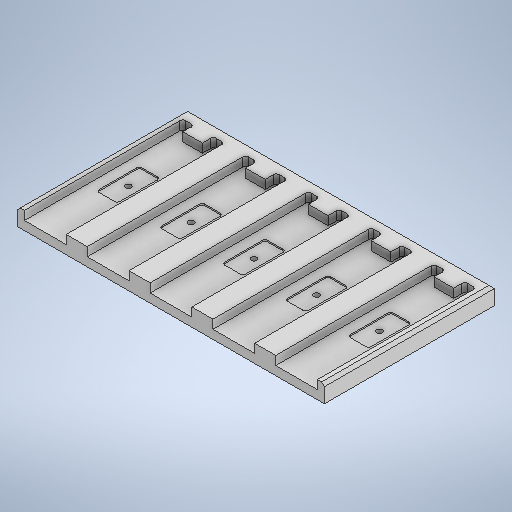
# Autodesk Inventor part: CROC Wirebonding Plate
Saved by Autodesk Inventor 2025 (Build 290162000, 162)
## iProperties
Created: 2025-05-07
Part Number: CROC Wirebonding Plate
Material: Generic
Document SubType Name: Modeling
Designer: Caleb Fangmeier
Density: 1 g/cm^3
Appearance: Default
Author: Caleb Fangmeier
Autodesk Inventor part; units mm, degrees
ref_plane "YZ Plane" through (0, 0, 0) normal (1, 0, 0) x (0, 1, 0)
ref_plane "XZ Plane" through (0, 0, 0) normal (0, 1, 0) x (-1, 0, 0)
ref_plane "XY Plane" through (0, 0, 0) normal (0, 0, 1) x (1, 0, 0)
sketch "Sketch1" plane through (0, 0, 0) normal (0, 1, 0) x (-1, 0, 0)
  line L0 (-111, 61.5) -> (111, 61.5)
  line L1 (111, 61.5) -> (111, -61.5)
  line L2 (111, -61.5) -> (-111, -61.5)
  line L3 (-111, -61.5) -> (-111, 61.5)
  line L4 (-111, 61.5) -> (111, -61.5) construction
  line L5 (111, 61.5) -> (-111, -61.5) construction
  point P0 (0, 0)
  dimension "d0" = 222
  dimension "d1" = 123
  constraints: 12 end point, 2 midpoint, 2 parallel, 1 horizontal, 1 perpendicular
  measures "d0" distance of L1.end L2.end
  measures "d1" distance of L0.end L1.end
extrude "Extrusion1" add sketch "Sketch1" along normal blind 12.7
sketch "Sketch2" plane through (0, 12.7, 0) normal (0, 1, 0) x (1, 0, 0)
  line L0 (-111, -61.5) -> (111, -61.5) projected
  line L1 (-106, -61.5) -> (-75.8, -61.5)
  line L2 (-75.8, -61.5) -> (-75.8, 45)
  line L3 (-75.8, 45) -> (-106, 45)
  line L4 (-106, 45) -> (-106, -61.5)
  line L5 (-111, 61.5) -> (-111, -61.5) projected
  line L6 (-106, 45) -> (-98, 45)
  line L7 (-98, 45) -> (-98, 51)
  line L8 (-100, 53) -> (-104, 53)
  line L9 (-106, 51) -> (-106, 45)
  line L10 (-75.8, 45) -> (-83.8, 45)
  line L11 (-83.8, 45) -> (-83.8, 51)
  line L12 (-81.8, 53) -> (-77.8, 53)
  line L13 (-75.8, 51) -> (-75.8, 45)
  arc A0 (-104, 53) -> (-106, 51) centre (-104, 51) ccw
  arc A1 (-98, 51) -> (-100, 53) centre (-100, 51) ccw
  arc A2 (-81.8, 53) -> (-83.8, 51) centre (-81.8, 51) ccw
  arc A3 (-75.8, 51) -> (-77.8, 53) centre (-77.8, 51) ccw
  line L14 (-60.55, -61.5) -> (-30.35, -61.5)
  line L15 (-30.35, -61.5) -> (-30.35, 45)
  arc A4 (-58.55, 53) -> (-60.55, 51) centre (-58.55, 51) ccw
  line L16 (-60.55, 51) -> (-60.55, 45)
  line L17 (-60.55, 45) -> (-60.55, -61.5)
  line L18 (-30.35, 45) -> (-60.55, 45)
  line L19 (-60.55, 45) -> (-52.55, 45)
  line L20 (-54.55, 53) -> (-58.55, 53)
  line L21 (-52.55, 45) -> (-52.55, 51)
  arc A5 (-52.55, 51) -> (-54.55, 53) centre (-54.55, 51) ccw
  line L22 (-38.35, 45) -> (-38.35, 51)
  arc A6 (-36.35, 53) -> (-38.35, 51) centre (-36.35, 51) ccw
  line L23 (-36.35, 53) -> (-32.35, 53)
  line L24 (-30.35, 45) -> (-38.35, 45)
  line L25 (-30.35, 51) -> (-30.35, 45)
  arc A7 (-30.35, 51) -> (-32.35, 53) centre (-32.35, 51) ccw
  line L26 (-15.1, -61.5) -> (15.1, -61.5)
  line L27 (15.1, -61.5) -> (15.1, 45)
  arc A8 (-13.1, 53) -> (-15.1, 51) centre (-13.1, 51) ccw
  line L28 (-15.1, 51) -> (-15.1, 45)
  line L29 (-15.1, 45) -> (-15.1, -61.5)
  line L30 (15.1, 45) -> (-15.1, 45)
  line L31 (-15.1, 45) -> (-7.1, 45)
  line L32 (-9.1, 53) -> (-13.1, 53)
  line L33 (-7.1, 45) -> (-7.1, 51)
  arc A9 (-7.1, 51) -> (-9.1, 53) centre (-9.1, 51) ccw
  line L34 (7.1, 45) -> (7.1, 51)
  arc A10 (9.1, 53) -> (7.1, 51) centre (9.1, 51) ccw
  line L35 (9.1, 53) -> (13.1, 53)
  line L36 (15.1, 45) -> (7.1, 45)
  line L37 (15.1, 51) -> (15.1, 45)
  arc A11 (15.1, 51) -> (13.1, 53) centre (13.1, 51) ccw
  line L38 (30.35, -61.5) -> (60.55, -61.5)
  line L39 (60.55, -61.5) -> (60.55, 45)
  arc A12 (32.35, 53) -> (30.35, 51) centre (32.35, 51) ccw
  line L40 (30.35, 51) -> (30.35, 45)
  line L41 (30.35, 45) -> (30.35, -61.5)
  line L42 (60.55, 45) -> (30.35, 45)
  line L43 (30.35, 45) -> (38.35, 45)
  line L44 (36.35, 53) -> (32.35, 53)
  line L45 (38.35, 45) -> (38.35, 51)
  arc A13 (38.35, 51) -> (36.35, 53) centre (36.35, 51) ccw
  line L46 (52.55, 45) -> (52.55, 51)
  arc A14 (54.55, 53) -> (52.55, 51) centre (54.55, 51) ccw
  line L47 (54.55, 53) -> (58.55, 53)
  line L48 (60.55, 45) -> (52.55, 45)
  line L49 (60.55, 51) -> (60.55, 45)
  arc A15 (60.55, 51) -> (58.55, 53) centre (58.55, 51) ccw
  line L50 (75.8, -61.5) -> (106, -61.5)
  line L51 (106, -61.5) -> (106, 45)
  arc A16 (77.8, 53) -> (75.8, 51) centre (77.8, 51) ccw
  line L52 (75.8, 51) -> (75.8, 45)
  line L53 (75.8, 45) -> (75.8, -61.5)
  line L54 (106, 45) -> (75.8, 45)
  line L55 (75.8, 45) -> (83.8, 45)
  line L56 (81.8, 53) -> (77.8, 53)
  line L57 (83.8, 45) -> (83.8, 51)
  arc A17 (83.8, 51) -> (81.8, 53) centre (81.8, 51) ccw
  line L58 (98, 45) -> (98, 51)
  arc A18 (100, 53) -> (98, 51) centre (100, 51) ccw
  line L59 (100, 53) -> (104, 53)
  line L60 (106, 45) -> (98, 45)
  line L61 (106, 51) -> (106, 45)
  arc A19 (106, 51) -> (104, 53) centre (104, 51) ccw
  point P0 (0, 0)
  point P1 (-98, 53)
  point P2 (-106, 53)
  point P3 (-83.8, 53)
  point P4 (-75.8, 53)
  point P5 (-60.55, 53)
  point P6 (-38.35, 53)
  point P7 (-52.55, 53)
  point P8 (-30.35, 53)
  point P9 (-15.1, 53)
  point P10 (7.1, 53)
  point P11 (-7.1, 53)
  point P12 (15.1, 53)
  point P13 (30.35, 53)
  point P14 (52.55, 53)
  point P15 (38.35, 53)
  point P16 (60.55, 53)
  point P17 (75.8, 53)
  point P18 (98, 53)
  point P19 (83.8, 53)
  point P20 (106, 53)
  dimension "d4" = 30.2
  dimension "d5" = 45
  dimension "d6" = 5
  dimension "d7" = 8
  dimension "d8" = 8
  dimension "d9" = 8
  dimension "d10" = 2
  dimension "d13" = 45.45
  constraints: 120 end point, 46 point on line, 40 point on circle, 20 centre point, 8 tangent, 6 parallel, 4 horizontal, 3 equal radius, 3 perpendicular, 1 collinear, 151 other
  measures "d4" distance of L2.end L3.end
  measures "d5" distance from line of L3 point (0, 0)
  measures "d6" distance between parallel lines of L5 L4
  measures "d7" distance of point (-106, 53) point (-98, 53)
  measures "d8" distance of point (-83.8, 53) point (-75.8, 53)
  measures "d9" distance between parallel lines of L8 L3
  measures "d10" radius of A0
  measures "d13" distance of L1.start L14.start
extrude "Extrusion2" cut sketch "Sketch2" against normal blind 6.35
sketch "Sketch3" plane through (0, 6.35, 0) normal (0, 1, 0) x (1, 0, 0)
  line L0 (-96.4, -17) -> (-85.4, -17)
  line L1 (-83.4, -15) -> (-83.4, 12)
  line L2 (-85.4, 14) -> (-96.4, 14)
  line L3 (-98.4, 12) -> (-98.4, -15)
  line L4 (-98, 45) -> (-83.8, 45) projected
  line L5 (-106, -61.5) -> (-106, 51) projected
  line L6 (-75.8, 51) -> (-75.8, -61.5) projected
  arc A0 (-96.4, 14) -> (-98.4, 12) centre (-96.4, 12) ccw
  arc A1 (-83.4, 12) -> (-85.4, 14) centre (-85.4, 12) ccw
  arc A2 (-98.4, -15) -> (-96.4, -17) centre (-96.4, -15) ccw
  arc A3 (-85.4, -17) -> (-83.4, -15) centre (-85.4, -15) ccw
  line L7 (-37.95, -15) -> (-37.95, 12)
  line L8 (-52.95, 12) -> (-52.95, -15)
  line L9 (-50.95, -17) -> (-39.95, -17)
  arc A4 (-52.95, -15) -> (-50.95, -17) centre (-50.95, -15) ccw
  arc A5 (-39.95, -17) -> (-37.95, -15) centre (-39.95, -15) ccw
  arc A6 (-50.95, 14) -> (-52.95, 12) centre (-50.95, 12) ccw
  arc A7 (-37.95, 12) -> (-39.95, 14) centre (-39.95, 12) ccw
  line L10 (-39.95, 14) -> (-50.95, 14)
  line L11 (7.5, -15) -> (7.5, 12)
  line L12 (-7.5, 12) -> (-7.5, -15)
  line L13 (-5.5, -17) -> (5.5, -17)
  arc A8 (-7.5, -15) -> (-5.5, -17) centre (-5.5, -15) ccw
  arc A9 (5.5, -17) -> (7.5, -15) centre (5.5, -15) ccw
  arc A10 (-5.5, 14) -> (-7.5, 12) centre (-5.5, 12) ccw
  arc A11 (7.5, 12) -> (5.5, 14) centre (5.5, 12) ccw
  line L14 (5.5, 14) -> (-5.5, 14)
  line L15 (52.95, -15) -> (52.95, 12)
  line L16 (37.95, 12) -> (37.95, -15)
  line L17 (39.95, -17) -> (50.95, -17)
  arc A12 (37.95, -15) -> (39.95, -17) centre (39.95, -15) ccw
  arc A13 (50.95, -17) -> (52.95, -15) centre (50.95, -15) ccw
  arc A14 (39.95, 14) -> (37.95, 12) centre (39.95, 12) ccw
  arc A15 (52.95, 12) -> (50.95, 14) centre (50.95, 12) ccw
  line L18 (50.95, 14) -> (39.95, 14)
  line L19 (98.4, -15) -> (98.4, 12)
  line L20 (83.4, 12) -> (83.4, -15)
  line L21 (85.4, -17) -> (96.4, -17)
  arc A16 (83.4, -15) -> (85.4, -17) centre (85.4, -15) ccw
  arc A17 (96.4, -17) -> (98.4, -15) centre (96.4, -15) ccw
  arc A18 (85.4, 14) -> (83.4, 12) centre (85.4, 12) ccw
  arc A19 (98.4, 12) -> (96.4, 14) centre (96.4, 12) ccw
  line L22 (96.4, 14) -> (85.4, 14)
  point P0 (0, 0)
  point P1 (-98.4, -17)
  point P2 (-83.4, 14)
  point P3 (-98.4, 14)
  point P4 (-90.9, -1.5)
  point P5 (-37.95, 14)
  point P6 (-52.95, 14)
  point P7 (-52.95, -17)
  point P8 (-45.45, -1.5)
  point P9 (7.5, 14)
  point P10 (-7.5, 14)
  point P11 (-7.5, -17)
  point P12 (0, -1.5)
  point P13 (52.95, 14)
  point P14 (37.95, 14)
  point P15 (37.95, -17)
  point P16 (45.45, -1.5)
  point P17 (98.4, 14)
  point P18 (83.4, 14)
  point P19 (83.4, -17)
  point P20 (90.9, -1.5)
  dimension "d20" = 31
  dimension "d21" = 15
  dimension "d22" = 31
  dimension "d23" = 30.2
  dimension "d24" = 7.6
  dimension "d25" = 2
  dimension "d26" = 15.5
  dimension "d27" = 7.5
  dimension "d30" = 45.45
  constraints: 40 end point, 40 point on circle, 30 point on line, 20 centre point, 8 tangent, 3 equal radius, 2 horizontal, 2 parallel, 1 perpendicular, 96 other
  measures "d20" distance between parallel lines of L4 L2
  measures "d21" distance of point (-83.4, 14) point (-98.4, 14)
  measures "d22" distance of point (-98.4, 14) point (-98.4, -17)
  measures "d23" distance between parallel lines of L5 L6
  measures "d24" distance between parallel lines of L5 L3
  measures "d25" radius of A0
  measures "d26" distance from line of L2 point (-90.9, -1.5)
  measures "d27" distance from line of point (-90.9, -1.5) L1
  measures "d30" distance of L1.start L7.start
extrude "Extrusion3" cut sketch "Sketch3" against normal blind 1
hole "Hole1" at (-90.9, 6.35, 1.5) at (-45.45, 6.35, 1.5) at (0, 6.35, 1.5) at (45.45, 6.35, 1.5) at (90.9, 6.35, 1.5) direction (0, -1, 0) diameter 4 end through all
chamfer "Chamfer1" distance 2 angle 45 3 edges at (-111, 12.7, 0) (0, 12.7, -61.5) (111, 12.7, 0)
equation "\"d8\" = d7"
equation "\"d24\" = -0.5 * d21 + 0.5 * d23"
body "Solid1"
